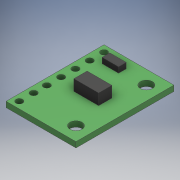
# Autodesk Inventor part: laser
Saved by Autodesk Inventor 2017 (Build 210142000, 142)
## iProperties
Part Number: laser
Material: Genérico
Document SubType Name: Modeling
Designer: Roberto
Density: 1 g/cm^3
Appearance: Valor por defecto
Author: Roberto
Autodesk Inventor part; units mm, degrees
ref_plane "YZ Plane" through (0, 0, 0) normal (1, 0, 0) x (0, 1, 0)
ref_plane "XZ Plane" through (0, 0, 0) normal (0, 1, 0) x (-1, 0, 0)
ref_plane "XY Plane" through (0, 0, 0) normal (0, 0, 1) x (1, 0, 0)
sketch "Boceto1" plane through (0, 0, 0) normal (0, 0, 1) x (1, 0, 0)
  line L0 (0, 1.78) -> (1.27, 1.78)
  line L1 (0.4602, 1.012) -> (0.4602, 0.772)
  line L2 (0.4602, 0.772) -> (0.9102, 0.772)
  line L3 (0.9102, 0.772) -> (0.9102, 1.012)
  line L4 (0.9102, 1.012) -> (0.4602, 1.012)
  line L5 (0, 1.78) -> (0, 0)
  line L6 (0, 0) -> (1.27, 0)
  line L7 (1.27, 0) -> (1.27, 1.78)
  line L8 (1.27, 1.78) -> (1.02, 1.78)
  circle A0 centre (1.02, 1.53) radius 0.11
  line L9 (0, 1.78) -> (0.12, 1.78)
  circle A1 centre (0.12, 1.66) radius 0.06
  circle A2 centre (0.12, 1.4) radius 0.06
  circle A3 centre (0.12, 1.14) radius 0.06
  circle A4 centre (0.12, 0.88) radius 0.06
  circle A5 centre (0.12, 0.62) radius 0.06
  circle A6 centre (0.12, 0.12) radius 0.06
  circle A7 centre (0.12, 0.38) radius 0.06
  line L10 (0.2802, 1.6043) -> (0.2802, 1.4643)
  line L11 (0.2802, 1.4643) -> (0.5802, 1.4643)
  line L12 (0.5802, 1.4643) -> (0.5802, 1.6043)
  line L13 (0.5802, 1.6043) -> (0.2802, 1.6043)
  circle A8 centre (1.02, 0.25) radius 0.11
  constraints: 28 end point, 9 centre point, 2 point on line
extrude "Extrusión1" add sketch "Boceto1" against normal blind 0.1 contours L0 L7 L6 L5 | L4 L3 L2 L1 | L13 L12 L11 L10
sketch "Boceto2" plane through (0, 0, 0) normal (0, 0, 1) x (1, 0, 0)
  line L0 (0, 1.78) -> (1.27, 1.78)
  line L1 (0.4602, 1.012) -> (0.4602, 0.772)
  line L2 (0.4602, 0.772) -> (0.9102, 0.772)
  line L3 (0.9102, 0.772) -> (0.9102, 1.012)
  line L4 (0.9102, 1.012) -> (0.4602, 1.012)
  line L5 (0, 1.78) -> (0, 0)
  line L6 (0, 0) -> (1.27, 0)
  line L7 (1.27, 0) -> (1.27, 1.78)
  line L8 (1.27, 1.78) -> (1.02, 1.78)
  circle A0 centre (1.02, 1.53) radius 0.11
  line L9 (0, 1.78) -> (0.12, 1.78)
  circle A1 centre (0.12, 1.66) radius 0.06
  circle A2 centre (0.12, 1.4) radius 0.06
  circle A3 centre (0.12, 1.14) radius 0.06
  circle A4 centre (0.12, 0.88) radius 0.06
  circle A5 centre (0.12, 0.62) radius 0.06
  circle A6 centre (0.12, 0.12) radius 0.06
  circle A7 centre (0.12, 0.38) radius 0.06
  line L10 (0.2802, 1.6043) -> (0.2802, 1.4643)
  line L11 (0.2802, 1.4643) -> (0.5802, 1.4643)
  line L12 (0.5802, 1.4643) -> (0.5802, 1.6043)
  line L13 (0.5802, 1.6043) -> (0.2802, 1.6043)
  circle A8 centre (1.02, 0.25) radius 0.11
  constraints: 28 end point, 9 centre point, 2 point on line
extrude "Extrusión2" add sketch "Boceto2" along normal blind 0.1 contours L13 L12 L11 L10
sketch "Boceto3" plane through (0, 0, 0) normal (0, 0, 1) x (1, 0, 0)
  line L0 (0, 1.78) -> (1.27, 1.78)
  line L1 (0.4602, 1.012) -> (0.4602, 0.772)
  line L2 (0.4602, 0.772) -> (0.9102, 0.772)
  line L3 (0.9102, 0.772) -> (0.9102, 1.012)
  line L4 (0.9102, 1.012) -> (0.4602, 1.012)
  line L5 (0, 1.78) -> (0, 0)
  line L6 (0, 0) -> (1.27, 0)
  line L7 (1.27, 0) -> (1.27, 1.78)
  line L8 (1.27, 1.78) -> (1.02, 1.78)
  circle A0 centre (1.02, 1.53) radius 0.11
  line L9 (0, 1.78) -> (0.12, 1.78)
  circle A1 centre (0.12, 1.66) radius 0.06
  circle A2 centre (0.12, 1.4) radius 0.06
  circle A3 centre (0.12, 1.14) radius 0.06
  circle A4 centre (0.12, 0.88) radius 0.06
  circle A5 centre (0.12, 0.62) radius 0.06
  circle A6 centre (0.12, 0.12) radius 0.06
  circle A7 centre (0.12, 0.38) radius 0.06
  line L10 (0.2802, 1.6043) -> (0.2802, 1.4643)
  line L11 (0.2802, 1.4643) -> (0.5802, 1.4643)
  line L12 (0.5802, 1.4643) -> (0.5802, 1.6043)
  line L13 (0.5802, 1.6043) -> (0.2802, 1.6043)
  circle A8 centre (1.02, 0.25) radius 0.11
  constraints: 28 end point, 9 centre point, 2 point on line
extrude "Extrusión3" add sketch "Boceto3" along normal blind 0.2 contours L4 L3 L2 L1
